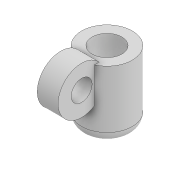
# Autodesk Inventor part: Landing_leg_shoe
Saved by Autodesk Inventor 2022 (Build 260153000, 153)
## iProperties
Created: 2022-07-01
Part Number: Landing_leg_shoe
Material: Generic
Document SubType Name: Modeling
Designer: dell
Density: 1 g/cm^3
Appearance: Default
Author: dell
Autodesk Inventor part; units mm, degrees
ref_plane "YZ Plane" through (0, 0, 0) normal (1, 0, 0) x (0, 1, 0)
ref_plane "XZ Plane" through (0, 0, 0) normal (0, 1, 0) x (-1, 0, 0)
ref_plane "XY Plane" through (0, 0, 0) normal (0, 0, 1) x (1, 0, 0)
sketch "Sketch1" plane through (0, 0, 0) normal (0, 1, 0) x (-1, 0, 0)
  circle A0 centre (0, 0) radius 2.85
  circle A1 centre (0, 0) radius 4.85
  dimension "d0" = 5.7
  dimension "d1" = 2
  constraints: 2 centre point, 1 coincident
  measures "d0" diameter of A0
  measures "d1" radial gap between concentric circles of A0 A1
extrude "Extrusion1" add sketch "Sketch1" along normal blind 10
sketch "Sketch2" plane through (0, 0, 0) normal (1, 0, 0) x (0, 1, 0)
  circle A0 centre (7, 6.85) radius 2
  circle A1 centre (7, 6.85) radius 4.5
  line L0 (10, -4.85) -> (10, 4.85) projected
  line L1 (0, -4.85) -> (0, 4.85) projected
  line L2 (0, 4.85) -> (10, 4.85) projected
  point P0 (0, 0)
  dimension "d4" = 4
  dimension "d5" = 9
  dimension "d6" = 7
  constraints: 2 centre point, 1 coincident, 1 tangent
  measures "d4" diameter of A0
  measures "d5" diameter of A1
  measures "d6" distance from line of L1 A0.centre
extrude "Extrusion2" add sketch "Sketch2" along normal mid plane 4
sketch "Sketch3" plane through (0, 0, 0) normal (0, -1, 0) x (1, 0, 0)
  circle A0 centre (0, 0) radius 4.85 projected
  circle A1 centre (0, 0) radius 2.85 projected
extrude "Extrusion3" add sketch "Sketch3" along normal blind 3 contours A0 | A1
fillet "Fillet1" radius 2 1 edges at (-4.85, -3, 0)
extrude "Extrusion4" cut sketch "Sketch1" along normal blind 100 contours A0
body "Solid1"
